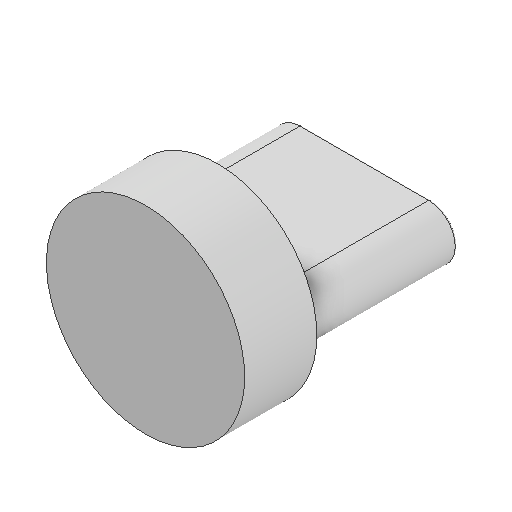
# Autodesk Inventor part: 磁吸頭
Saved by Autodesk Inventor 2025.2 (Build 292293000, 293)
## iProperties
Created: 2025-07-22
Part Number: 磁吸頭
Material: 一般
Document SubType Name: Modeling
Designer: jna1j
Density: 1 g/cm^3
Appearance: 預設
Author: jna1j
Autodesk Inventor part; units mm, degrees
ref_plane "YZ Plane" through (0, 0, 0) normal (1, 0, 0) x (0, 1, 0)
ref_plane "XZ Plane" through (0, 0, 0) normal (0, 1, 0) x (-1, 0, 0)
ref_plane "XY Plane" through (0, 0, 0) normal (0, 0, 1) x (1, 0, 0)
sketch "草圖1" plane through (0, 0, 0) normal (0, 0, 1) x (1, 0, 0)
  circle A0 centre (0, 0) radius 4.53
  dimension "d0" = 9.06
  constraints: 1 centre point, 1 coincident
  measures "d0" diameter of A0
extrude "擠出1" add sketch "草圖1" along normal blind 3.3
sketch "草圖2" plane through (0, 0, 0) normal (0, 0, -1) x (-1, 0, 0)
  line L0 (2.9402, 1.1992) -> (-2.9402, 1.1992)
  line L1 (-2.9402, -1.2408) -> (2.9402, -1.2408)
  arc A0 (-2.9402, 1.1992) -> (-2.9402, -1.2408) centre (-2.9402, -0.0208) ccw
  arc A1 (2.9402, -1.2408) -> (2.9402, 1.1992) centre (2.9402, -0.0208) ccw
  line L2 (-4.16, 0) -> (4.16, 0) construction
  arc A2 (2.9402, -0.7408) -> (2.9402, 0.6992) centre (2.9402, -0.0208) ccw
  line L3 (2.9402, 0.6992) -> (-2.9402, 0.6992)
  arc A3 (-2.9402, 0.6992) -> (-2.9402, -0.7408) centre (-2.9402, -0.0208) ccw
  line L4 (-2.9402, -0.7408) -> (2.9402, -0.7408)
  point P0 (0, 0)
  point P1 (0, 0)
  dimension "d3" = 8.32
  dimension "d5" = 2.44
  dimension "d6" = 0.5
  constraints: 10 end point, 10 point on circle, 4 centre point, 2 horizontal, 2 parallel, 1 coincident, 1 midpoint, 3 other
  measures "d3" distance of L2.start L2.end
  measures "d5" distance between parallel lines of L0 L1
  measures "d6" distance between parallel lines of L1 L4
extrude "擠出2" add sketch "草圖2" along normal blind 6.8
fillet "圓角1" radius 0.1 8 edges at (4.1602, -0.0208, -6.8) (0, -1.2408, -6.8) (-4.1602, -0.0208, -6.8) (0, 1.1992, -6.8) (-3.6602, -0.0208, -6.8) (0, -0.7408, -6.8) (3.6602, -0.0208, -6.8) (0, 0.6992, -6.8)
